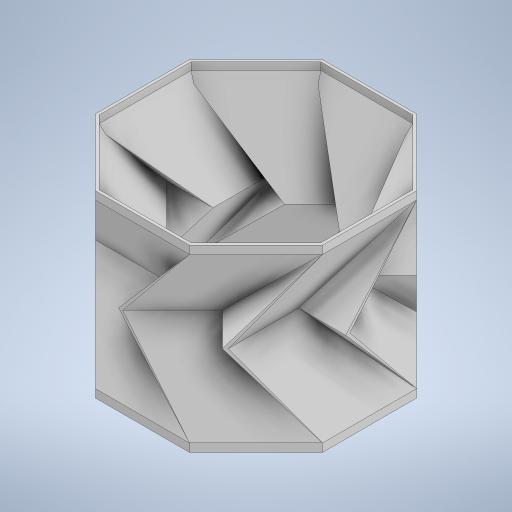
# Autodesk Inventor part: OV-PAM_half_scale_1F_0.4
Saved by Autodesk Inventor 2024 (Build 280153000, 153)
## iProperties
Created: 2023-06-16
Part Number: OV-PAM_half_scale_1F_0.4
Material: 일반
Document SubType Name: Modeling
Designer: jsw
Density: 1 g/cm^3
Appearance: 기본값
Author: jsw
Autodesk Inventor part; units mm, degrees
ref_plane "YZ Plane" through (0, 0, 0) normal (1, 0, 0) x (0, 1, 0)
ref_plane "XZ Plane" through (0, 0, 0) normal (0, 1, 0) x (-1, 0, 0)
ref_plane "XY Plane" through (0, 0, 0) normal (0, 0, 1) x (1, 0, 0)
sketch "스케치1" plane through (0, 0, 0) normal (0, 1, 0) x (-1, 0, 0)
  line L0 (-16.295942, 6.75) -> (-6.75, 16.295942)
  line L1 (-6.75, 16.295942) -> (6.75, 16.295942)
  line L2 (6.75, 16.295942) -> (16.295942, 6.75)
  line L3 (16.295942, 6.75) -> (16.295942, -6.75)
  line L4 (16.295942, -6.75) -> (6.75, -16.295942)
  line L5 (6.75, -16.295942) -> (-6.75, -16.295942)
  line L6 (-6.75, -16.295942) -> (-16.295942, -6.75)
  line L7 (-16.295942, -6.75) -> (-16.295942, 6.75)
  line L8 (-6.915685, 16.695942) -> (6.915685, 16.695942)
  line L9 (6.915685, 16.695942) -> (16.695942, 6.915685)
  line L10 (16.695942, 6.915685) -> (16.695942, -6.915685)
  line L11 (16.695942, -6.915685) -> (6.915685, -16.695942)
  line L12 (6.915685, -16.695942) -> (-6.915685, -16.695942)
  line L13 (-6.915685, -16.695942) -> (-16.695942, -6.915685)
  line L14 (-16.695942, -6.915685) -> (-16.695942, 6.915685)
  line L15 (-16.695942, 6.915685) -> (-6.915685, 16.695942)
  point P0 (0, 0)
  point P1 (0, 0)
  point P2 (0, 0)
  dimension "d0" = 13.5
  dimension "d2" = 0.4
  constraints: 32 end point, 2 coincident, 2 horizontal, 34 other
  measures "d0" distance of L0.end L1.end
  measures "d2" distance between parallel lines of L10 L3
extrude "돌출2" add sketch "스케치1" along normal blind 12 contours L0 L1 L2 L3 L4 L5 L6 L7 | L8 L9 L10 L11 L12 L13 L14 L15
ref_plane "작업 평면2" through (16.695942, 0, 6.915685) normal (-0.8660254, -0.5, 0) x (0, 0, -1)
sketch "스케치3" plane through (16.695942, 0, 6.915685) normal (1, 0, 0) x (0, 0, -1)
  line L0 (0, 0) -> (0, 12)
  line L1 (0, 12) -> (13.831371, 12)
  line L2 (0, 0) -> (13.831371, 0)
  line L3 (13.831371, 0) -> (13.831371, 12)
  line L4 (13.831371, 12) -> (0, 12)
  line L5 (0, 12) -> (0, 0)
  line L6 (0, 12) -> (-7.304723, 12)
  line L7 (-9.780256, 12) -> (0, 12)
  line L8 (0, 0) -> (-7.304723, 12)
  line L9 (13.831371, 12) -> (6.915685, 12)
  line L10 (3.415685, 12) -> (13.831371, 0)
  point P0 (6.915685, 0)
  dimension "d17" = 121.33
  dimension "d53" = 3.5
  constraints: 16 end point, 6 midpoint, 2 parallel, 2 point on line, 1 horizontal, 1 perpendicular
  measures "d17" angle of L8 L2
  measures "d53" distance of L10.start point (6.916, 12)
extrude "돌출4" cut sketch "스케치3" against normal up to surface contours L8 L6 L0 | L0 L1 L10 L2 surface through (16.695942, 0, 6.915685) normal (-0.8660254, -0.5, 0)
pattern_circular "원형 패턴1" count 8 over 360 about axis through (0, -10, 0) along (0, 1, 0) of "돌출4"
mirror "미러5" about plane through (0, 12, 0) normal (0, 1, 0) of "돌출2", "돌출4", "원형 패턴1"
sketch "스케치9" plane through (-6.915685, 24, -16.695942) normal (0, 1, 0) x (1, 0, 0)
  line L0 (23.611627, -23.611627) -> (23.611627, -9.780256)
  line L1 (23.611627, -9.780256) -> (13.831371, 0)
  line L2 (13.831371, 0) -> (0, 0)
  line L3 (0, 0) -> (-9.780256, -9.780256)
  line L4 (-9.780256, -9.780256) -> (-9.780256, -23.611627)
  line L5 (-9.780256, -23.611627) -> (0, -33.391883)
  line L6 (0, -33.391883) -> (13.831371, -33.391883)
  line L7 (13.831371, -33.391883) -> (23.611627, -23.611627)
  point P0 (6.915685, -16.695942)
extrude "돌출8" add sketch "스케치9" along normal blind 1.2
sketch "스케치10" plane through (0, 0, 0) normal (0, -1, 0) x (1, 0, 0)
  line L0 (16.695942, 6.915685) -> (16.695942, -6.915685)
  line L1 (6.915685, 16.695942) -> (16.695942, 6.915685)
  line L2 (-6.915685, 16.695942) -> (6.915685, 16.695942)
  line L3 (-16.695942, 6.915685) -> (-6.915685, 16.695942)
  line L4 (-16.695942, -6.915685) -> (-16.695942, 6.915685)
  line L5 (-6.915685, -16.695942) -> (-16.695942, -6.915685)
  line L6 (6.915685, -16.695942) -> (-6.915685, -16.695942)
  line L7 (16.695942, -6.915685) -> (6.915685, -16.695942)
  point P0 (0, 0)
extrude "돌출9" add sketch "스케치10" along normal blind 1.2
shell "쉘6" thickness 0.4 removed faces 2 at (-0.954857, 25.2, 2.305228) at (5.565314, -1.2, -2.305228)
